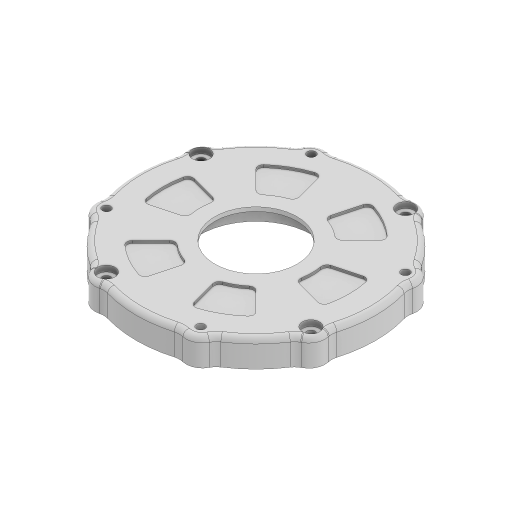
# Autodesk Inventor part: tapa
Saved by Autodesk Inventor 2024.3 (Build 283343000, 343)
## iProperties
Created: 2025-03-05
Part Number: tapa
Material: Generic
Document SubType Name: Modeling
Designer: danie
Density: 1 g/cm^3
Appearance: Default
Author: danie
Autodesk Inventor part; units mm, degrees
ref_plane "YZ Plane" through (0, 0, 0) normal (1, 0, 0) x (0, 1, 0)
ref_plane "XZ Plane" through (0, 0, 0) normal (0, 1, 0) x (-1, 0, 0)
ref_plane "XY Plane" through (0, 0, 0) normal (0, 0, 1) x (1, 0, 0)
sketch "Block1" plane through (0, 0, 0) normal (0, 0, 1) x (1, 0, 0)
  arc A0 (57.749739, -25.97075) -> (44.669035, -38.975982) centre (82.263491, -63.707681) ccw
  arc A1 (57.749739, -25.97075) -> (59.814236, -23.688549) centre (54.481239, -20.939159) ccw
  arc A2 (66.536977, -20.601106) -> (59.814236, -23.688549) centre (65.147233, -26.437938) ccw
  arc A3 (66.536977, -20.601106) -> (69.613401, -20.522322) centre (67.926722, -14.764274) ccw
  circle A4 centre (64.557017, -25.152775) radius 1.5875
  arc A5 (39.078132, -51.057591) -> (39.138869, -47.907444) centre (33.320084, -49.370912) ccw
  circle A6 centre (43.759974, -45.889735) radius 1.5875
  arc A7 (42.307048, -41.061199) -> (39.138869, -47.907444) centre (44.957654, -46.443976) ccw
  arc A8 (42.307048, -41.061199) -> (44.669035, -38.975982) centre (39.656441, -35.678422) ccw
  arc A9 (94.913581, -20.522322) -> (69.613401, -20.522322) centre (82.263491, -63.707681) ccw
  circle A10 centre (100.081436, -25.204164) radius 1.5875
  arc A11 (104.909973, -23.751238) -> (106.99519, -26.113225) centre (110.292749, -21.100631) ccw
  arc A12 (104.909973, -23.751238) -> (98.063728, -20.583059) centre (99.527196, -26.401844) ccw
  arc A13 (94.913581, -20.522322) -> (98.063728, -20.583059) centre (96.600259, -14.764274) ccw
  arc A14 (39.093337, -79.383085) -> (39.041714, -76.232775) centre (33.27881, -77.902788) ccw
  arc A15 (39.078132, -51.057591) -> (39.041714, -76.232775) centre (82.263491, -63.707681) ccw
  arc A16 (125.433645, -48.032277) -> (122.285287, -41.176894) centre (119.619118, -46.55198) ccw
  arc A17 (119.929342, -39.084852) -> (122.285287, -41.176894) centre (124.951455, -35.801809) ccw
  arc A18 (119.929342, -39.084852) -> (106.99519, -26.113225) centre (82.263491, -63.707681) ccw
  arc A19 (39.093337, -79.383085) -> (42.241695, -86.238467) centre (44.907864, -80.863382) ccw
  circle A20 centre (43.708585, -81.414155) radius 1.5875
  arc A21 (44.59764, -88.330509) -> (57.531792, -101.302136) centre (82.263491, -63.707681) ccw
  arc A22 (44.59764, -88.330509) -> (42.241695, -86.238467) centre (39.575526, -91.613553) ccw
  circle A23 centre (64.445545, -102.211198) radius 1.5875
  arc A24 (59.617009, -103.664124) -> (57.531792, -101.302136) centre (54.234232, -106.31473) ccw
  arc A25 (59.617009, -103.664124) -> (66.463254, -106.832302) centre (64.999786, -101.013517) ccw
  arc A26 (69.613401, -106.89304) -> (66.463254, -106.832302) centre (67.926722, -112.651088) ccw
  arc A27 (125.433645, -48.032277) -> (125.485268, -51.182586) centre (131.248171, -49.512574) ccw
  circle A28 centre (120.818397, -46.001207) radius 1.5875
  arc A29 (125.416427, -76.467934) -> (125.485268, -51.182586) centre (82.263491, -63.707681) ccw
  arc A30 (69.613401, -106.89304) -> (94.788585, -106.929458) centre (82.263491, -63.707681) ccw
  arc A31 (125.416427, -76.467934) -> (125.339628, -79.585276) centre (131.170152, -78.169301) ccw
  circle A32 centre (120.767008, -81.525626) radius 1.5875
  arc A33 (122.189822, -86.369095) -> (125.339628, -79.585276) centre (119.509104, -81.001251) ccw
  arc A34 (122.189822, -86.369095) -> (119.857946, -88.43938) centre (124.87054, -91.736939) ccw
  arc A35 (97.9063, -106.869634) -> (94.788585, -106.929458) centre (96.458598, -112.692361) ccw
  circle A36 centre (99.969965, -102.262587) radius 1.5875
  arc A37 (106.79012, -101.436244) -> (119.857946, -88.43938) centre (82.263491, -63.707681) ccw
  arc A38 (106.79012, -101.436244) -> (104.707169, -103.756812) centre (110.060337, -106.466719) ccw
  arc A39 (97.9063, -106.869634) -> (104.707169, -103.756812) centre (99.354001, -101.046906) ccw
  point P0 (82.255304, -63.715982)
  point P1 (82.263491, -63.707681)
sketch "Sketch1" plane through (0, 0, 0) normal (0, 1, 0) x (-1, 0, 0)
  circle A0 centre (0, 0) radius 21.1
  circle A1 centre (0, 0) radius 45
  dimension "d0" = 42.2
  dimension "d1" = 90
  constraints: 2 centre point, 2 coincident
  measures "d0" diameter of A0
  measures "d1" diameter of A1
extrude "Extrusion1" add sketch "Sketch1" along normal blind 8
sketch "Sketch2" plane through (0, 8, 0) normal (0, 1, 0) x (1, 0, 0)
  circle A0 centre (0, 0) radius 21.1 projected
  circle A1 centre (0, 0) radius 15
  dimension "d4" = 30
  constraints: 1 centre point, 1 coincident
  measures "d4" diameter of A1
extrude "Extrusion2" add sketch "Sketch2" against normal blind 2
sketch "Sketch5" plane through (0, 8, 0) normal (0, 1, 0) x (1, 0, 0)
  circle A0 centre (0, 0) radius 15 projected
  circle A1 centre (0, 0) radius 45 projected
  line L0 (-35, -35) -> (35, -35)
  line L1 (35, -35) -> (35, 35)
  line L2 (35, 35) -> (-35, 35)
  line L3 (-35, 35) -> (-35, -35)
  line L4 (-35, -35) -> (35, 35) construction
  line L5 (35, -35) -> (-35, 35) construction
  line L6 (-30, -30) -> (30, -30)
  line L7 (30, -30) -> (30, 30)
  line L8 (30, 30) -> (-30, 30)
  line L9 (-30, 30) -> (-30, -30)
  line L10 (-30, -30) -> (30, 30) construction
  line L11 (30, -30) -> (-30, 30) construction
  circle A2 centre (-30, 30) radius 1.5875
  circle A3 centre (30, 30) radius 1.5875
  circle A4 centre (-30, -30) radius 1.5875
  circle A5 centre (30, -30) radius 1.5875
  point P0 (35, -28.284271)
  point P1 (28.284271, -35)
  point P2 (-35, -28.284271)
  point P3 (-28.284271, -35)
  point P4 (28.284271, 35)
  point P5 (35, 28.284271)
  point P6 (-35, 28.284271)
  point P7 (-28.284271, 35)
  dimension "d24" = 70
  dimension "d25" = 70
  dimension "d26" = 60
  dimension "d27" = 3.175
  dimension "d30" = 60
  dimension "d33" = 60
  constraints: 24 end point, 4 centre point, 4 midpoint, 4 parallel, 3 horizontal, 2 perpendicular, 1 coincident, 1 point on line, 1 vertical, 6 other
  measures "d24" distance between parallel lines of L1 L3
  measures "d25" distance between parallel lines of L0 L2
  measures "d26" distance of L6.end L7.end
  measures "d27" diameter of A2
  measures "d30" distance of A2.centre A3.centre
  measures "d33" distance of A2.centre A4.centre
sketch "Sketch7" plane through (0, 8, 0) normal (0, 1, 0) x (1, 0, 0)
  circle A0 centre (0, 0) radius 15
  circle A1 centre (0, 0) radius 45
  circle A2 centre (0, 0) radius 12.65009
  arc A3 (-24.513752, 37.736931) -> (-37.594455, 24.731699) centre (0, 0) ccw
  arc A4 (-24.513752, 37.736931) -> (-22.449255, 40.019132) centre (-27.782252, 42.768522) ccw
  arc A5 (-15.726513, 43.106575) -> (-22.449255, 40.019132) centre (-17.116258, 37.269742) ccw
  arc A6 (-15.726513, 43.106575) -> (-12.65009, 43.185359) centre (-14.336769, 48.943407) ccw
  circle A7 centre (-17.706474, 38.554906) radius 1.5875
  arc A8 (-43.185359, 12.65009) -> (-43.124622, 15.800237) centre (-48.943407, 14.336769) ccw
  circle A9 centre (-38.503517, 17.817946) radius 1.5875
  arc A10 (-39.956443, 22.646482) -> (-43.124622, 15.800237) centre (-37.305836, 17.263705) ccw
  arc A11 (-39.956443, 22.646482) -> (-37.594455, 24.731699) centre (-42.607049, 28.029259) ccw
  arc A12 (12.65009, 43.185359) -> (-12.65009, 43.185359) centre (0, 0) ccw
  circle A13 centre (17.817946, 38.503517) radius 1.5875
  arc A14 (22.646482, 39.956443) -> (24.731699, 37.594455) centre (28.029259, 42.607049) ccw
  arc A15 (22.646482, 39.956443) -> (15.800237, 43.124622) centre (17.263705, 37.305836) ccw
  arc A16 (12.65009, 43.185359) -> (15.800237, 43.124622) centre (14.336769, 48.943407) ccw
  arc A17 (-43.170154, -15.675404) -> (-43.221777, -12.525095) centre (-48.984681, -14.195107) ccw
  arc A18 (-43.185359, 12.65009) -> (-43.221777, -12.525095) centre (0, 0) ccw
  arc A19 (43.170154, 15.675404) -> (40.021796, 22.530787) centre (37.355627, 17.155701) ccw
  arc A20 (37.665851, 24.622828) -> (40.021796, 22.530787) centre (42.687964, 27.905872) ccw
  arc A21 (37.665851, 24.622828) -> (24.731699, 37.594455) centre (0, 0) ccw
  arc A22 (-43.170154, -15.675404) -> (-40.021796, -22.530787) centre (-37.355627, -17.155701) ccw
  circle A23 centre (-38.554906, -17.706474) radius 1.5875
  arc A24 (-37.665851, -24.622828) -> (-24.731699, -37.594455) centre (0, 0) ccw
  arc A25 (-37.665851, -24.622828) -> (-40.021796, -22.530787) centre (-42.687964, -27.905872) ccw
  circle A26 centre (-17.817946, -38.503517) radius 1.5875
  arc A27 (-22.646482, -39.956443) -> (-24.731699, -37.594455) centre (-28.029259, -42.607049) ccw
  arc A28 (-22.646482, -39.956443) -> (-15.800237, -43.124622) centre (-17.263705, -37.305836) ccw
  arc A29 (-12.65009, -43.185359) -> (-15.800237, -43.124622) centre (-14.336769, -48.943407) ccw
  arc A30 (43.170154, 15.675404) -> (43.221777, 12.525095) centre (48.984681, 14.195107) ccw
  circle A31 centre (38.554906, 17.706474) radius 1.5875
  arc A32 (43.152937, -12.760253) -> (43.221777, 12.525095) centre (0, 0) ccw
  arc A33 (-12.65009, -43.185359) -> (12.525095, -43.221777) centre (0, 0) ccw
  arc A34 (43.152937, -12.760253) -> (43.076137, -15.877595) centre (48.906662, -14.46162) ccw
  circle A35 centre (38.503517, -17.817946) radius 1.5875
  arc A36 (39.926331, -22.661415) -> (43.076137, -15.877595) centre (37.245613, -17.293571) ccw
  arc A37 (39.926331, -22.661415) -> (37.594455, -24.731699) centre (42.607049, -28.029259) ccw
  arc A38 (15.642809, -43.161953) -> (12.525095, -43.221777) centre (14.195107, -48.984681) ccw
  circle A39 centre (17.706474, -38.554906) radius 1.5875
  arc A40 (24.526629, -37.728563) -> (37.594455, -24.731699) centre (0, 0) ccw
  arc A41 (24.526629, -37.728563) -> (22.443678, -40.049131) centre (27.796846, -42.759038) ccw
  arc A42 (15.642809, -43.161953) -> (22.443678, -40.049131) centre (17.090511, -37.339225) ccw
  point P0 (-12.65009, -43.185359)
  point P1 (24.526629, -37.728563)
  point P2 (12.525095, -43.221777)
  point P3 (43.152937, -12.760253)
  point P4 (37.594455, -24.731699)
  point P5 (37.665851, 24.622828)
  point P6 (43.221777, 12.525095)
  point P7 (12.65009, 43.185359)
  point P8 (24.731699, 37.594455)
  point P9 (-24.513752, 37.736931)
  point P10 (-12.65009, 43.185359)
  point P11 (-43.185359, 12.65009)
  point P12 (-37.594455, 24.731699)
  point P13 (-37.665851, -24.622828)
  point P14 (-43.221777, -12.525095)
  constraints: 1 centre point, 1 concentric, 1 other
extrude "Extrusion6" add sketch "Sketch7" against normal up to surface (8 mm away) contours A1 A20 A19 A30 | A34 A36 A37 A1 | A1 A16 A15 A14 | A41 A42 A38 A1 | A1 A4 A5 A6 | A29 A28 A27 A1 | A1 A8 A10 A11 | A25 A22 A17 A1
extrude "Extrusion7" cut sketch "Sketch7" against normal blind 10 contours A7 | A9 | A13 | A23 | A26 | A31 | A35 | A39
sketch "Sketch3" plane through (0, 8, 0) normal (0, 1, 0) x (1, 0, 0)
  circle A0 centre (0, 0) radius 15 projected
  circle A1 centre (0, 0) radius 45 projected
  circle A2 centre (0, 0) radius 41
  circle A3 centre (-41, 0) radius 1.75
  dimension "d7" = 82
  dimension "d8" = 3.5
  constraints: 1 centre point, 1 coincident, 1 horizontal alignment, 2 other
  measures "d8" diameter of A3
sketch "Sketch4" plane through (0, 8, 0) normal (0, 1, 0) x (1, 0, 0)
  circle A0 centre (0, 0) radius 15
  circle A1 centre (-41, 0) radius 1.75
  circle A2 centre (-20.5, -35.507042) radius 1.75
  circle A3 centre (20.5, -35.507042) radius 1.75
  circle A4 centre (41, 0) radius 1.75
  circle A5 centre (20.5, 35.507042) radius 1.75
  circle A6 centre (-20.5, 35.507042) radius 1.75
  circle A7 centre (0, 0) radius 43
move faces "Move1" translate (0, 2.2, 0) faces at (32.487316, 8, -6.847781)
sketch "Sketch8" plane through (0, 0, 0) normal (0, -1, 0) x (1, 0, 0)
  circle A0 centre (17.706474, 38.554906) radius 1.5875
  circle A1 centre (-17.706474, -38.554906) radius 1.5875
  circle A2 centre (17.817946, -38.503517) radius 1.5875
  circle A3 centre (-17.817946, 38.503517) radius 1.5875
  circle A4 centre (38.503517, 17.817946) radius 1.5875
  circle A5 centre (-38.503517, -17.817946) radius 1.5875
  circle A6 centre (38.554906, -17.706474) radius 1.5875
  circle A7 centre (-38.554906, 17.706474) radius 1.5875
  arc A8 (-43.221777, 12.525095) -> (-43.185359, -12.65009) centre (0, 0) ccw
  arc A9 (-43.124622, -15.800237) -> (-43.185359, -12.65009) centre (-48.943407, -14.336769) ccw
  arc A10 (-43.124622, -15.800237) -> (-39.956443, -22.646482) centre (-37.305836, -17.263705) ccw
  arc A11 (-37.594455, -24.731699) -> (-39.956443, -22.646482) centre (-42.607049, -28.029259) ccw
  arc A12 (-37.594455, -24.731699) -> (-24.513752, -37.736931) centre (0, 0) ccw
  arc A13 (-22.449255, -40.019132) -> (-24.513752, -37.736931) centre (-27.782252, -42.768522) ccw
  arc A14 (-22.449255, -40.019132) -> (-15.726513, -43.106575) centre (-17.116258, -37.269742) ccw
  arc A15 (-12.65009, -43.185359) -> (-15.726513, -43.106575) centre (-14.336769, -48.943407) ccw
  arc A16 (-12.65009, -43.185359) -> (12.65009, -43.185359) centre (0, 0) ccw
  arc A17 (15.800237, -43.124622) -> (12.65009, -43.185359) centre (14.336769, -48.943407) ccw
  arc A18 (15.800237, -43.124622) -> (22.646482, -39.956443) centre (17.263705, -37.305836) ccw
  arc A19 (24.731699, -37.594455) -> (22.646482, -39.956443) centre (28.029259, -42.607049) ccw
  arc A20 (24.731699, -37.594455) -> (37.665851, -24.622828) centre (0, 0) ccw
  arc A21 (40.021796, -22.530787) -> (37.665851, -24.622828) centre (42.687964, -27.905872) ccw
  arc A22 (40.021796, -22.530787) -> (43.170154, -15.675404) centre (37.355627, -17.155701) ccw
  arc A23 (43.221777, -12.525095) -> (43.170154, -15.675404) centre (48.984681, -14.195107) ccw
  arc A24 (43.221777, -12.525095) -> (43.152937, 12.760253) centre (0, 0) ccw
  arc A25 (43.076137, 15.877595) -> (43.152937, 12.760253) centre (48.906662, 14.46162) ccw
  arc A26 (43.076137, 15.877595) -> (39.926331, 22.661415) centre (37.245613, 17.293571) ccw
  arc A27 (37.594455, 24.731699) -> (39.926331, 22.661415) centre (42.607049, 28.029259) ccw
  arc A28 (37.594455, 24.731699) -> (24.526629, 37.728563) centre (0, 0) ccw
  arc A29 (22.443678, 40.049131) -> (24.526629, 37.728563) centre (27.796846, 42.759038) ccw
  arc A30 (22.443678, 40.049131) -> (15.642809, 43.161953) centre (17.090511, 37.339225) ccw
  arc A31 (12.525095, 43.221777) -> (15.642809, 43.161953) centre (14.195107, 48.984681) ccw
  arc A32 (12.525095, 43.221777) -> (-12.65009, 43.185359) centre (0, 0) ccw
  arc A33 (-15.800237, 43.124622) -> (-12.65009, 43.185359) centre (-14.336769, 48.943407) ccw
  arc A34 (-15.800237, 43.124622) -> (-22.646482, 39.956443) centre (-17.263705, 37.305836) ccw
  arc A35 (-24.731699, 37.594455) -> (-22.646482, 39.956443) centre (-28.029259, 42.607049) ccw
  arc A36 (-24.731699, 37.594455) -> (-37.665851, 24.622828) centre (0, 0) ccw
  arc A37 (-40.021796, 22.530787) -> (-37.665851, 24.622828) centre (-42.687964, 27.905872) ccw
  arc A38 (-40.021796, 22.530787) -> (-43.170154, 15.675404) centre (-37.355627, 17.155701) ccw
  arc A39 (-43.221777, 12.525095) -> (-43.170154, 15.675404) centre (-48.984681, 14.195107) ccw
  circle A40 centre (0, 0) radius 21.1
  circle A41 centre (0, 0) radius 31.25
  dimension "d52" = 62.5
  constraints: 1 centre point, 1 coincident
  measures "d52" diameter of A41
extrude "Extrusion8" cut sketch "Sketch8" against normal blind 1.5 contours A41
move faces "Move2" translate (0, 2.7, 0) faces at (-18.717, 6, 2.879765)
sketch "Sketch9" plane through (0, 10.2, 0) normal (0, 1, 0) x (1, 0, 0)
  circle A0 centre (17.706474, -38.554906) radius 1.5875
  circle A1 centre (-17.706474, 38.554906) radius 1.5875
  circle A2 centre (17.817946, 38.503517) radius 1.5875
  circle A3 centre (-17.817946, -38.503517) radius 1.5875
  circle A4 centre (38.503517, -17.817946) radius 1.5875
  circle A5 centre (-38.503517, 17.817946) radius 1.5875
  circle A6 centre (38.554906, 17.706474) radius 1.5875
  circle A7 centre (-38.554906, -17.706474) radius 1.5875
  circle A8 centre (0, 0) radius 15
  arc A9 (-43.185359, 12.65009) -> (-43.221777, -12.525095) centre (0, 0) ccw
  arc A10 (-43.170154, -15.675404) -> (-43.221777, -12.525095) centre (-48.984681, -14.195107) ccw
  arc A11 (-43.170154, -15.675404) -> (-40.021796, -22.530787) centre (-37.355627, -17.155701) ccw
  arc A12 (-37.665851, -24.622828) -> (-40.021796, -22.530787) centre (-42.687964, -27.905872) ccw
  arc A13 (-37.665851, -24.622828) -> (-24.731699, -37.594455) centre (0, 0) ccw
  arc A14 (-22.646482, -39.956443) -> (-24.731699, -37.594455) centre (-28.029259, -42.607049) ccw
  arc A15 (-22.646482, -39.956443) -> (-15.800237, -43.124622) centre (-17.263705, -37.305836) ccw
  arc A16 (-12.65009, -43.185359) -> (-15.800237, -43.124622) centre (-14.336769, -48.943407) ccw
  arc A17 (-12.65009, -43.185359) -> (12.525095, -43.221777) centre (0, 0) ccw
  arc A18 (15.642809, -43.161953) -> (12.525095, -43.221777) centre (14.195107, -48.984681) ccw
  arc A19 (15.642809, -43.161953) -> (22.443678, -40.049131) centre (17.090511, -37.339225) ccw
  arc A20 (24.526629, -37.728563) -> (22.443678, -40.049131) centre (27.796846, -42.759038) ccw
  arc A21 (24.526629, -37.728563) -> (37.594455, -24.731699) centre (0, 0) ccw
  arc A22 (39.926331, -22.661415) -> (37.594455, -24.731699) centre (42.607049, -28.029259) ccw
  arc A23 (39.926331, -22.661415) -> (43.076137, -15.877595) centre (37.245613, -17.293571) ccw
  arc A24 (43.152937, -12.760253) -> (43.076137, -15.877595) centre (48.906662, -14.46162) ccw
  arc A25 (43.152937, -12.760253) -> (43.221777, 12.525095) centre (0, 0) ccw
  arc A26 (43.170154, 15.675404) -> (43.221777, 12.525095) centre (48.984681, 14.195107) ccw
  arc A27 (43.170154, 15.675404) -> (40.021796, 22.530787) centre (37.355627, 17.155701) ccw
  arc A28 (37.665851, 24.622828) -> (40.021796, 22.530787) centre (42.687964, 27.905872) ccw
  arc A29 (37.665851, 24.622828) -> (24.731699, 37.594455) centre (0, 0) ccw
  arc A30 (22.646482, 39.956443) -> (24.731699, 37.594455) centre (28.029259, 42.607049) ccw
  arc A31 (22.646482, 39.956443) -> (15.800237, 43.124622) centre (17.263705, 37.305836) ccw
  arc A32 (12.65009, 43.185359) -> (15.800237, 43.124622) centre (14.336769, 48.943407) ccw
  arc A33 (12.65009, 43.185359) -> (-12.65009, 43.185359) centre (0, 0) ccw
  arc A34 (-15.726513, 43.106575) -> (-12.65009, 43.185359) centre (-14.336769, 48.943407) ccw
  arc A35 (-15.726513, 43.106575) -> (-22.449255, 40.019132) centre (-17.116258, 37.269742) ccw
  arc A36 (-24.513752, 37.736931) -> (-22.449255, 40.019132) centre (-27.782252, 42.768522) ccw
  arc A37 (-24.513752, 37.736931) -> (-37.594455, 24.731699) centre (0, 0) ccw
  arc A38 (-39.956443, 22.646482) -> (-37.594455, 24.731699) centre (-42.607049, 28.029259) ccw
  arc A39 (-39.956443, 22.646482) -> (-43.124622, 15.800237) centre (-37.305836, 17.263705) ccw
  arc A40 (-43.185359, 12.65009) -> (-43.124622, 15.800237) centre (-48.943407, 14.336769) ccw
  circle A41 centre (0, 0) radius 15.5
  dimension "d58" = 31
  constraints: 1 centre point, 1 coincident
  measures "d58" diameter of A41
extrude "Extrusion9" cut sketch "Sketch9" against normal up to surface (1.5 mm away) contours A41
sketch "Sketch10" plane through (0, 10.2, 0) normal (0, 1, 0) x (1, 0, 0)
  circle A0 centre (0, 0) radius 15.5
  circle A1 centre (17.706474, -38.554906) radius 1.5875
  circle A2 centre (-17.706474, 38.554906) radius 1.5875
  circle A3 centre (17.817946, 38.503517) radius 1.5875
  circle A4 centre (-17.817946, -38.503517) radius 1.5875
  circle A5 centre (38.503517, -17.817946) radius 1.5875
  circle A6 centre (-38.503517, 17.817946) radius 1.5875
  circle A7 centre (38.554906, 17.706474) radius 1.5875
  circle A8 centre (-38.554906, -17.706474) radius 1.5875
  arc A9 (-43.185359, 12.65009) -> (-43.221777, -12.525095) centre (0, 0) ccw
  arc A10 (-43.170154, -15.675404) -> (-43.221777, -12.525095) centre (-48.984681, -14.195107) ccw
  arc A11 (-43.170154, -15.675404) -> (-40.021796, -22.530787) centre (-37.355627, -17.155701) ccw
  arc A12 (-37.665851, -24.622828) -> (-40.021796, -22.530787) centre (-42.687964, -27.905872) ccw
  arc A13 (-37.665851, -24.622828) -> (-24.731699, -37.594455) centre (0, 0) ccw
  arc A14 (-22.646482, -39.956443) -> (-24.731699, -37.594455) centre (-28.029259, -42.607049) ccw
  arc A15 (-22.646482, -39.956443) -> (-15.800237, -43.124622) centre (-17.263705, -37.305836) ccw
  arc A16 (-12.65009, -43.185359) -> (-15.800237, -43.124622) centre (-14.336769, -48.943407) ccw
  arc A17 (-12.65009, -43.185359) -> (12.525095, -43.221777) centre (0, 0) ccw
  arc A18 (15.642809, -43.161953) -> (12.525095, -43.221777) centre (14.195107, -48.984681) ccw
  arc A19 (15.642809, -43.161953) -> (22.443678, -40.049131) centre (17.090511, -37.339225) ccw
  arc A20 (24.526629, -37.728563) -> (22.443678, -40.049131) centre (27.796846, -42.759038) ccw
  arc A21 (24.526629, -37.728563) -> (37.594455, -24.731699) centre (0, 0) ccw
  arc A22 (39.926331, -22.661415) -> (37.594455, -24.731699) centre (42.607049, -28.029259) ccw
  arc A23 (39.926331, -22.661415) -> (43.076137, -15.877595) centre (37.245613, -17.293571) ccw
  arc A24 (43.152937, -12.760253) -> (43.076137, -15.877595) centre (48.906662, -14.46162) ccw
  arc A25 (43.152937, -12.760253) -> (43.221777, 12.525095) centre (0, 0) ccw
  arc A26 (43.170154, 15.675404) -> (43.221777, 12.525095) centre (48.984681, 14.195107) ccw
  arc A27 (43.170154, 15.675404) -> (40.021796, 22.530787) centre (37.355627, 17.155701) ccw
  arc A28 (37.665851, 24.622828) -> (40.021796, 22.530787) centre (42.687964, 27.905872) ccw
  arc A29 (37.665851, 24.622828) -> (24.731699, 37.594455) centre (0, 0) ccw
  arc A30 (22.646482, 39.956443) -> (24.731699, 37.594455) centre (28.029259, 42.607049) ccw
  arc A31 (22.646482, 39.956443) -> (15.800237, 43.124622) centre (17.263705, 37.305836) ccw
  arc A32 (12.65009, 43.185359) -> (15.800237, 43.124622) centre (14.336769, 48.943407) ccw
  arc A33 (12.65009, 43.185359) -> (-12.65009, 43.185359) centre (0, 0) ccw
  arc A34 (-15.726513, 43.106575) -> (-12.65009, 43.185359) centre (-14.336769, 48.943407) ccw
  arc A35 (-15.726513, 43.106575) -> (-22.449255, 40.019132) centre (-17.116258, 37.269742) ccw
  arc A36 (-24.513752, 37.736931) -> (-22.449255, 40.019132) centre (-27.782252, 42.768522) ccw
  arc A37 (-24.513752, 37.736931) -> (-37.594455, 24.731699) centre (0, 0) ccw
  arc A38 (-39.956443, 22.646482) -> (-37.594455, 24.731699) centre (-42.607049, 28.029259) ccw
  arc A39 (-39.956443, 22.646482) -> (-43.124622, 15.800237) centre (-37.305836, 17.263705) ccw
  arc A40 (-43.185359, 12.65009) -> (-43.124622, 15.800237) centre (-48.943407, 14.336769) ccw
hole "Hole2" at (-38.503517, 10.2, -17.817946) at (17.817946, 10.2, -38.503517) at (-17.817946, 10.2, 38.503517) at (38.503517, 10.2, 17.817946) direction (0, -1, 0) diameter 3.175 depth 15 tip angle 118 counterbore diameter 6.5 counterbore depth 2.2
fillet "Fillet1" radius 2 32 edges at (31.8658, 10.2, -31.7737) (23.5313, 10.2, -38.6361) (19.7835, 10.2, -42.7511) (14.2211, 10.2, -42.9445) (0, 10.2, -45) (-14.1832, 10.2, -42.9454) (-19.6203, 10.2, -42.7222) (-23.3327, 10.2, -38.7434) (-31.7276, 10.2, -31.9117) (-38.6361, 10.2, -23.5313) (-42.7511, 10.2, -19.7835) (-42.9445, 10.2, -14.2211) (-45, 10.2, -0.0651) (-42.9855, 10.2, 14.0968) (-42.8081, 10.2, 19.6598) (-38.704, 10.2, 23.4194) (-31.8658, 10.2, 31.7737) (-23.5313, 10.2, 38.6361) (-19.7835, 10.2, 42.7511) (-14.2211, 10.2, 42.9445) (-0.0651, 10.2, 45) (14.08, 10.2, 42.9858) (19.5876, 10.2, 42.7949) (23.3318, 10.2, 38.7512) (31.7331, 10.2, 31.9063) (38.6235, 10.2, 23.5424) (42.6876, 10.2, 19.8204) (42.9085, 10.2, 14.3138) (44.9998, 10.2, 0.1225) (42.9855, 10.2, -14.0968) (42.8081, 10.2, -19.6598) (38.704, 10.2, -23.4194)
sketch "Sketch11" plane through (0, 10.2, 0) normal (0, 1, 0) x (1, 0, 0)
  circle A0 centre (0, 0) radius 21.1
  circle A1 centre (-38.554906, -17.706474) radius 1.5875
  circle A2 centre (38.554906, 17.706474) radius 1.5875
  circle A3 centre (-17.706474, 38.554906) radius 1.5875
  circle A4 centre (17.706474, -38.554906) radius 1.5875
  circle A5 centre (0, 0) radius 15.5
  arc A6 (12.087864, 41.26601) -> (15.846255, 41.087107) centre (14.336769, 48.943407) ccw
  arc A7 (12.087864, 41.26601) -> (-12.087864, 41.26601) centre (0, 0) ccw
  arc A8 (-16.189762, 41.160964) -> (-12.087864, 41.26601) centre (-14.336769, 48.943407) ccw
  arc A9 (-16.189762, 41.160964) -> (-20.671589, 39.102669) centre (-17.116258, 37.269742) ccw
  arc A10 (-23.424252, 36.059734) -> (-20.671589, 39.102669) centre (-27.782252, 42.768522) ccw
  arc A11 (-23.424252, 36.059734) -> (-35.923591, 23.632512) centre (0, 0) ccw
  arc A12 (-38.67275, 21.063536) -> (-35.923591, 23.632512) centre (-42.607049, 28.029259) ccw
  arc A13 (-41.087107, 15.846255) -> (-38.67275, 21.063536) centre (-38.503517, 17.817946) ccw
  arc A14 (-41.26601, 12.087864) -> (-41.087107, 15.846255) centre (-48.943407, 14.336769) ccw
  arc A15 (-41.26601, 12.087864) -> (-41.300809, -11.968424) centre (0, 0) ccw
  arc A16 (-41.231978, -16.168836) -> (-41.300809, -11.968424) centre (-48.984681, -14.195107) ccw
  arc A17 (-41.231978, -16.168836) -> (-39.133073, -20.739091) centre (-37.355627, -17.155701) ccw
  arc A18 (-35.991813, -23.52848) -> (-39.133073, -20.739091) centre (-42.687964, -27.905872) ccw
  arc A19 (-35.991813, -23.52848) -> (-23.632512, -35.923591) centre (0, 0) ccw
  arc A20 (-21.063536, -38.67275) -> (-23.632512, -35.923591) centre (-28.029259, -42.607049) ccw
  arc A21 (-15.846255, -41.087107) -> (-21.063536, -38.67275) centre (-17.817946, -38.503517) ccw
  arc A22 (-12.087864, -41.26601) -> (-15.846255, -41.087107) centre (-14.336769, -48.943407) ccw
  arc A23 (-12.087864, -41.26601) -> (11.968424, -41.300809) centre (0, 0) ccw
  arc A24 (16.125376, -41.221043) -> (11.968424, -41.300809) centre (14.195107, -48.984681) ccw
  arc A25 (16.125376, -41.221043) -> (20.659289, -39.145829) centre (17.090511, -37.339225) ccw
  arc A26 (23.436557, -36.051738) -> (20.659289, -39.145829) centre (27.796846, -42.759038) ccw
  arc A27 (23.436557, -36.051738) -> (35.923591, -23.632512) centre (0, 0) ccw
  arc A28 (38.67275, -21.063536) -> (35.923591, -23.632512) centre (42.607049, -28.029259) ccw
  arc A29 (41.011177, -15.750547) -> (38.67275, -21.063536) centre (38.503517, -17.817946) ccw
  arc A30 (41.235028, -12.193131) -> (41.011177, -15.750547) centre (48.906662, -14.46162) ccw
  arc A31 (41.235028, -12.193131) -> (41.300809, 11.968424) centre (0, 0) ccw
  arc A32 (41.231978, 16.168836) -> (41.300809, 11.968424) centre (48.984681, 14.195107) ccw
  arc A33 (41.231978, 16.168836) -> (39.133073, 20.739091) centre (37.355627, 17.155701) ccw
  arc A34 (35.991813, 23.52848) -> (39.133073, 20.739091) centre (42.687964, 27.905872) ccw
  arc A35 (35.991813, 23.52848) -> (23.632512, 35.923591) centre (0, 0) ccw
  arc A36 (21.063536, 38.67275) -> (23.632512, 35.923591) centre (28.029259, 42.607049) ccw
  arc A37 (15.846255, 41.087107) -> (21.063536, 38.67275) centre (17.817946, 38.503517) ccw
  circle A38 centre (0, 0) radius 35
  line L0 (-21.1, 0) -> (-35, 0)
  line L1 (0, 0) -> (-33.807404, 9.058667)
  line L2 (0, 0) -> (-33.807404, -9.058667)
  point P0 (-20.381035, -5.461082)
  point P1 (-20.381035, 5.461082)
  dimension "d69" = 70
  dimension "d70" = 15
  dimension "d71" = 15
  dimension "d43" = 42.42641
  dimension "d44" = 45
  constraints: 6 end point, 3 point on circle, 1 centre point, 1 coincident, 1 horizontal, 2 other
  measures "d69" diameter of A38
  measures "d70" angle of L0 L2
  measures "d71" angle of L1 L0
extrude "Extrusion10" cut sketch "Sketch11" against normal blind 1 contours A0 L0 A38 L1 | L2 A38 L0 A0
fillet "Fillet3" radius 2 4 edges at (-20.381, 9.7, 5.4611) (-20.381, 9.7, -5.4611) (-33.8074, 9.7, 9.0587) (-33.8074, 9.7, -9.0587)
pattern_circular "Circular Pattern3" count 6 over 360 about axis through (0, 10.2, 0) along (0, -1, 0) of "Extrusion10", "Fillet3"
body "Solid1"
